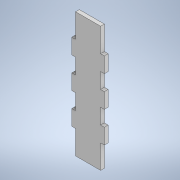
# Autodesk Inventor part: Sides_2
Saved by Autodesk Inventor 2020 (Build 240168000, 168)
## iProperties
Created: 2020-12-28
Part Number: Sides_2
Material: Generic
Document SubType Name: Modeling
Designer: solar
Density: 1 g/cm^3
Appearance: Default
Author: solar
Autodesk Inventor part; units mm, degrees
ref_plane "YZ Plane" through (0, 0, 0) normal (1, 0, 0) x (0, 1, 0)
ref_plane "XZ Plane" through (0, 0, 0) normal (0, 1, 0) x (-1, 0, 0)
ref_plane "XY Plane" through (0, 0, 0) normal (0, 0, 1) x (1, 0, 0)
sketch "Sketch1" plane through (0, 0, 0) normal (0, 0, 1) x (1, 0, 0)
  line L0 (-34, 0) -> (-34, 100)
  line L1 (-54, -12.375) -> (-60, -12.375)
  line L2 (-60, 37.125) -> (-54, 37.125)
  line L3 (-54, 61.875) -> (-60, 61.875)
  line L4 (-60, 12.375) -> (-54, 12.375)
  line L5 (-60, -37.125) -> (-54, -37.125)
  line L6 (-54, -61.875) -> (-60, -61.875)
  line L7 (-54, 61.875) -> (-54, 100)
  line L8 (-54, 37.125) -> (-54, 12.375)
  line L9 (-60, 37.125) -> (-60, 61.875)
  line L10 (-54, -12.375) -> (-54, -37.125)
  line L11 (-54, 100) -> (-34, 100)
  line L12 (-60, -61.875) -> (-60, -37.125)
  line L13 (-60, -12.375) -> (-60, 12.375)
  line L14 (-54, -61.875) -> (-54, -100)
  line L15 (-34, -100) -> (-54, -100)
  line L16 (-14, -12.375) -> (-8, -12.375)
  line L17 (-8, 37.125) -> (-14, 37.125)
  line L18 (-14, 61.875) -> (-8, 61.875)
  line L19 (-8, 12.375) -> (-14, 12.375)
  line L20 (-8, -37.125) -> (-14, -37.125)
  line L21 (-14, -61.875) -> (-8, -61.875)
  line L22 (-14, 61.875) -> (-14, 100)
  line L23 (-14, 37.125) -> (-14, 12.375)
  line L24 (-8, 37.125) -> (-8, 61.875)
  line L25 (-14, -12.375) -> (-14, -37.125)
  line L26 (-14, 100) -> (-34, 100)
  line L27 (-8, -61.875) -> (-8, -37.125)
  line L28 (-8, -12.375) -> (-8, 12.375)
  line L29 (-14, -61.875) -> (-14, -100)
  line L30 (-34, -100) -> (-14, -100)
  constraints: 62 end point, 14 symmetric about line, 2 horizontal
extrude "Extrusion1" add sketch "Sketch1" along normal blind 6
body "Solid1"
